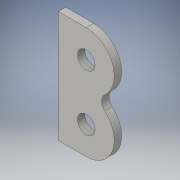
# Autodesk Inventor part: Nathan_RobotArm_B
Saved by Autodesk Inventor 2016 (Build 200138000, 138)
## iProperties
Created: 2017-03-30
Part Number: Nathan_RobotArm_B
Material: Generic
Document SubType Name: Modeling
Designer: brandn
Density: 1 g/cm^3
Appearance: Default
Author: brandn
Autodesk Inventor part; units mm, degrees
ref_plane "YZ Plane" through (0, 0, 0) normal (1, 0, 0) x (0, 1, 0)
ref_plane "XZ Plane" through (0, 0, 0) normal (0, 1, 0) x (-1, 0, 0)
ref_plane "XY Plane" through (0, 0, 0) normal (0, 0, 1) x (1, 0, 0)
sketch "Sketch1" plane through (0, 0, 0) normal (0, 0, 1) x (1, 0, 0)
  line L0 (0, 0) -> (9.525, 0)
  line L1 (9.525, 38.1) -> (0, 38.1)
  line L2 (0, 38.1) -> (0, 0)
  arc A0 (15.8252, 21.4312) -> (9.525, 38.1) centre (9.525, 28.575) ccw
  arc A1 (9.525, 0) -> (15.8252, 16.6687) centre (9.525, 9.525) ccw
  circle A2 centre (9.525, 28.575) radius 3
  circle A3 centre (9.525, 9.525) radius 3
  arc A4 (15.8252, 21.4312) -> (15.8252, 16.6687) centre (17.9253, 19.05) ccw
  point P0 (19.05, 19.05)
  dimension "d2" = 19.05
  dimension "d3" = 38.1
  dimension "d4" = 9.525
  dimension "d5" = 9.525
  dimension "d6" = 9.525
  dimension "d9" = 90
  dimension "d11" = 6
  dimension "d12" = 6
  dimension "d13" = 9.525
  dimension "d14" = 9.525
  dimension "d15" = 9.525
  dimension "d16" = 9.525
  dimension "d17" = 3.175
  dimension "d18" = 9.525
  constraints: 6 end point, 6 point on circle, 5 centre point, 3 tangent, 1 horizontal, 1 parallel
  measures "d3" distance of L0.start L1.end
  measures "d4" radius of A0
  measures "d5" distance from line of L2 A0.centre
  measures "d6" radius of A1
  measures "d9" angle of L2 L1
  measures "d11" diameter of A2
  measures "d12" diameter of A3
  measures "d13" distance from line of L2 A2.centre
  measures "d14" distance of L1.start A2.centre
  measures "d15" distance from line of L2 A3.centre
  measures "d16" distance of L0.end A3.centre
  measures "d17" radius of A4
  measures "d18" vertical distance of A4.centre A2.centre
extrude "Extrusion1" add sketch "Sketch1" along normal blind 2.54
body "Solid1"
